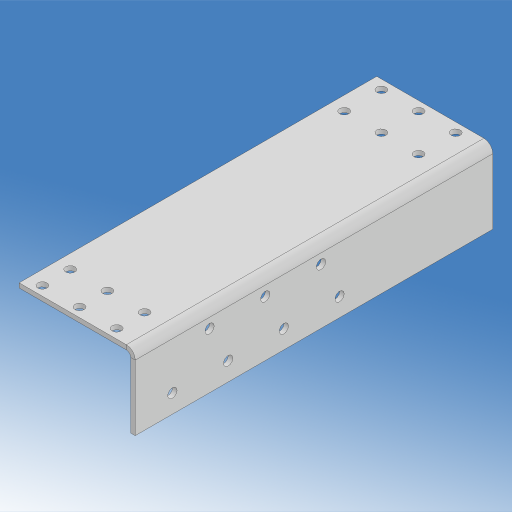
# Autodesk Inventor part: MainDriveMotorToPlateConnector
Saved by Autodesk Inventor 2024 (Build 280153000, 153)
## iProperties
Created: 2024-04-02
Part Number: MainDriveMotorToPlateConnector
Material: Generic
Document SubType Name: Sheet Metal
Designer: seene
Density: 1 g/cm^3
Sheet Metal Rule: Default
Appearance: Default
Author: seene
Autodesk Inventor part; units mm, degrees
ref_plane "YZ Plane" through (0, 0, 0) normal (1, 0, 0) x (0, 1, 0)
ref_plane "XZ Plane" through (0, 0, 0) normal (0, 1, 0) x (-1, 0, 0)
ref_plane "XY Plane" through (0, 0, 0) normal (0, 0, 1) x (1, 0, 0)
sketch "Sketch1" plane through (0, 0, 0) normal (0, 1, 0) x (-1, 0, 0)
  line L0 (0, 0) -> (79.375, 0)
  line L1 (79.375, 0) -> (79.375, -244.475)
  line L2 (79.375, -244.475) -> (0, -244.475)
  line L3 (0, -244.475) -> (0, 0)
  circle A0 centre (69.85, -6.35) radius 3.175
  circle A1 centre (69.85, -25.4) radius 3.175
  circle A2 centre (44.45, -6.35) radius 3.175
  circle A3 centre (44.45, -25.4) radius 3.175
  circle A4 centre (19.05, -6.35) radius 3.175
  circle A5 centre (19.05, -25.4) radius 3.175
  circle A6 centre (69.85, -212.725) radius 3.175
  circle A7 centre (69.85, -238.125) radius 3.175
  circle A8 centre (44.45, -212.725) radius 3.175
  circle A9 centre (44.45, -238.125) radius 3.175
  circle A10 centre (19.05, -212.725) radius 3.175
  circle A11 centre (19.05, -238.125) radius 3.175
  dimension "d0" = 79.375
  dimension "d2" = 6.35
  dimension "d3" = 6.35
  dimension "d4" = 9.525
  dimension "d7" = 19.05
  dimension "d10" = 25.4
  dimension "d15" = 25.4
  dimension "d18" = 25.4
  dimension "d21" = 206.375
  dimension "d22" = 6.35
  measures "d0" distance of L1.end L2.end
  measures "d2" diameter of A0
  measures "d3" distance from line of A0.centre L0
  measures "d4" distance from line of L1 A0.centre
  measures "d7" distance of A0.centre A1.centre
  measures "d10" distance of A0.centre A2.centre
  measures "d15" distance of A6.centre A7.centre
  measures "d18" distance of A6.centre A8.centre
  measures "d21" distance of A6.centre A0.centre
  measures "d22" distance from line of L2 A7.centre
extrude "Plate1" add sketch "Sketch1" along normal blind 3.048
sketch "Sketch2" plane through (-3.048, 3.048, 0) normal (1, 0, 0) x (0, 1, 0)
  line L0 (0, -244.475) -> (0, 0)
  line L1 (0, 0) -> (-50.8, 0)
  line L2 (-50.8, 0) -> (-50.8, -244.475)
  line L3 (-50.8, -244.475) -> (0, -244.475)
  constraints: 6 end point, 1 horizontal, 1 perpendicular, 1 vertical
edge flange "Flange1" height 50.8 angle 90 thickness 3.048 bend radius 3.048 thickness toward (1, 0, 0) relief straight relief width 3.048 relief depth 1.524 edges at (0, 0, -122.2375) wall of the first edge with corners at (-3.048, 3.048, -244.475) (-3.048, 3.048, 0) (-3.048, -47.752, 0) (-3.048, -47.752, -244.475)
bend "Bend1"
corner "Corner1"
sketch "Sketch3" plane through (0, -47.752, 0) normal (1, 0, 0) x (0, 0, -1)
  circle A0 centre (50.8, 37.9611) radius 3.175
  circle A1 centre (25.4, 12.5611) radius 3.175
  line L0 (0, 0) -> (0, 44.704) projected
  line L1 (244.475, 0) -> (0, 0) projected
  circle A2 centre (63.5, 12.5611) radius 3.175
  circle A3 centre (101.6, 12.5611) radius 3.175
  circle A4 centre (139.7, 12.5611) radius 3.175
  circle A5 centre (88.9, 37.9611) radius 3.175
  circle A6 centre (127, 37.9611) radius 3.175
  point P0 (0, 47.752)
  dimension "d34" = 6.35
  dimension "d35" = 25.4
  dimension "d36" = 25.4
  dimension "d37" = 25.4
  dimension "d40" = 38.1
  dimension "d47" = 38.1
  constraints: 7 centre point, 2 horizontal, 1 equal radius, 10 other
  measures "d34" diameter of A0
  measures "d35" horizontal distance of A0.centre A1.centre
  measures "d36" horizontal distance of A0.centre A1.centre
  measures "d37" distance from line of A1.centre L0
  measures "d40" distance of A1.centre A2.centre
  measures "d47" distance of A0.centre A5.centre
extrude "Cut1" cut sketch "Sketch3" against normal blind 3.048
equation "\"d52\" = Thickness"
equation "\"d23\" = Thickness"
equation "\"d24\" = BendReliefWidth"
equation "\"d25\" = BendReliefDepth"
equation "\"d26\" = MinimumRemnant"
equation "\"d27\" = TransitionRadius"
equation "\"d30\" = BendRadius"
equation "\"d31\" = CornerReliefSize"
equation "\"d32\" = GapSize"
equation "\"d33\" = JacobiRadiusSize"
equation "\"BendRadius\" = Thickness"
equation "\"BendReliefWidth\" = Thickness"
equation "\"BendReliefDepth\" = 0.5 * Thickness"
equation "\"CornerReliefSize\" = 4 * Thickness"
equation "\"MinimumRemnant\" = 2 * Thickness"
equation "\"TransitionRadius\" = BendRadius"
equation "\"JacobiRadiusSize\" = BendRadius"
equation "\"GapSize\" = Thickness"
equation "\"Thickness\" = 3.048"
body "Solid1"
